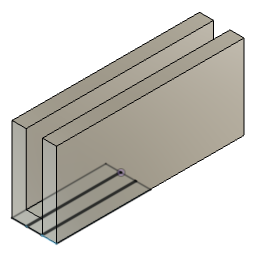
Table_Spacer (Autodesk Fusion 360 design; units mm, degrees)
Autodesk Fusion 360 part; units mm, degrees
sketch "Sketch1" plane through (0, 0, 0) normal (0, 0, 1) x (1, 0, 0)
  line L0 (0, 0) -> (3, 0)
  line L1 (3, 0) -> (3, -20)
  line L2 (3, -20) -> (0, -20)
  line L3 (0, -20) -> (0, 0)
  line L4 (3, 0) -> (3.25, 0)
  line L5 (3.25, 0) -> (3.25, -20)
  line L6 (3.25, -20) -> (3, -20)
  line L7 (3, -20) -> (3, 0)
  line L8 (0, 0) -> (-0.25, 0)
  line L9 (-0.25, 0) -> (-0.25, -20)
  line L10 (-0.25, -20) -> (0, -20)
  line L11 (0, -20) -> (0, 0)
  line L12 (3.25, 0) -> (6.25, 0)
  line L13 (6.25, 0) -> (6.25, -20.0231)
  line L14 (6.25, -20.0231) -> (3.25, -20.0231)
  line L15 (3.25, -20.0231) -> (3.25, 0)
  line L16 (-0.25, 0) -> (-3.25, 0)
  line L17 (-3.25, 0) -> (-3.25, -20)
  line L18 (-3.25, -20) -> (-0.25, -20)
  line L19 (-0.25, -20) -> (-0.25, 0)
  dimension "d1" = 3
  dimension "d2" = 20
  dimension "d3" = 0.25
  dimension "d4" = 0.25
  dimension "d5" = 3
  dimension "d6" = 3
  dimension "d7" = 20
  constraint horizontal L0
  constraint vertical L1
  constraint horizontal L2
  constraint vertical L3
  constraint coincident L0.start L3.end
  constraint horizontal L4
  constraint vertical L5
  constraint horizontal L6
  constraint vertical L7
  constraint horizontal L8
  constraint vertical L9
  constraint horizontal L10
  constraint vertical L11
  constraint horizontal L12
  constraint vertical L13
  constraint horizontal L14
  constraint vertical L15
  constraint horizontal L16
  constraint vertical L17
  constraint horizontal L18
  constraint vertical L19
  measures "d1" distance of L0.start L0.end
  measures "d2" distance of L0.start L2.end
  measures "d3" distance of L0.end L4.end
  measures "d4" distance of L0.start L8.end
  measures "d5" distance of L4.end L12.end
  measures "d6" distance of L8.end L16.end
  measures "d7" distance of L8.end L9.end
extrude "Extrude1" add sketch "Sketch1" along normal blind 3 contours L0 L1 L2 L3 L7 L11 | L3 L8 L9 L10 L11 L19 | L1 L4 L5 L6 L7 L15
extrude "Extrude2" add sketch "Sketch1" along normal blind 18 contours L9 L16 L17 L18 L19 | L5 L12 L13 L14 L15
extrude "Extrude3" add 1 faces at (5.25, -6.6744, 18) along direction (0, 0, 1) blind 15
extrude "Extrude4" cut 1 faces at (5.25, -6.6744, 33) along direction (0, 0, -1) blind 15
extrude "Extrude5" add 1 faces at (-2.25, 0, 7) along direction (0, 1, 0) blind 20
